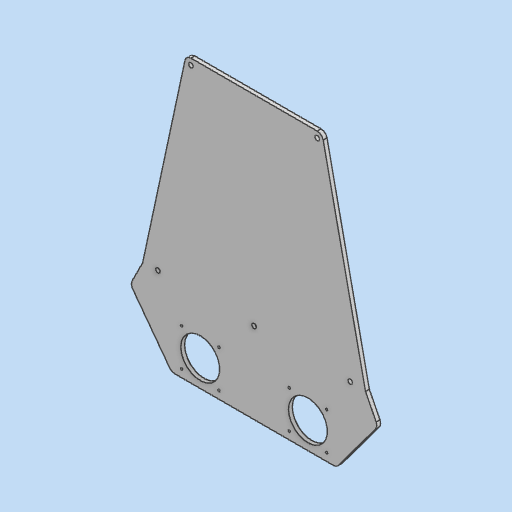
# Autodesk Inventor part: ChestFrontPanel
Saved by Autodesk Inventor 2025.2 (Build 292293000, 293)
## iProperties
Created: 2025-09-23
Part Number: ChestFrontPanel
Material: Generic
Document SubType Name: Sheet Metal
Designer: valer
Density: 1 g/cm^3
Sheet Metal Rule: Default_mm
Appearance: Default
Author: valer
Autodesk Inventor part; units mm, degrees
ref_plane "YZ Plane" through (0, 0, 0) normal (1, 0, 0) x (0, 1, 0)
ref_plane "XZ Plane" through (0, 0, 0) normal (0, 1, 0) x (-1, 0, 0)
ref_plane "XY Plane" through (0, 0, 0) normal (0, 0, 1) x (1, 0, 0)
sketch "Base" plane through (0, 0, 0) normal (0, 0, 1) x (1, 0, 0)
  line L0 (-341.7653, 0) -> (341.7653, 0) construction
  line L1 (0, -75.5138) -> (0, 453.0828) construction
  line L2 (183.676, 264.154) -> (223.6199, 230.6371) construction
  arc A0 (180.154, 267.676) -> (183.676, 264.154) centre (202.0437, 286.0437) ccw construction
  line L3 (105.6111, 356.5128) -> (180.154, 267.676) construction
  arc A1 (105.6111, 356.5128) -> (69.1282, 373.525) centre (69.1282, 325.9) ccw construction
  line L4 (-69.1282, 373.525) -> (69.1282, 373.525) construction
  arc A2 (231.2425, 165.7605) -> (223.6199, 230.6371) centre (193.0071, 194.1542) ccw construction
  line L5 (231.2425, 165.7605) -> (183.8243, 101.9065) construction
  line L6 (0, 373.525) -> (69.1282, 373.525) construction
  line L7 (183.8243, 101.9065) -> (108.1482, 0) construction
  line L8 (-183.676, 264.154) -> (-223.6199, 230.6371) construction
  arc A3 (-183.676, 264.154) -> (-180.154, 267.676) centre (-202.0437, 286.0437) ccw construction
  line L9 (-105.6111, 356.5128) -> (-180.154, 267.676) construction
  arc A4 (-69.1282, 373.525) -> (-105.6111, 356.5128) centre (-69.1282, 325.9) ccw construction
  arc A5 (-223.6199, 230.6371) -> (-231.2425, 165.7605) centre (-193.0071, 194.1542) ccw construction
  line L10 (-231.2425, 165.7605) -> (-183.8243, 101.9065) construction
  line L11 (0, 373.525) -> (-69.1282, 373.525) construction
  line L12 (-183.8243, 101.9065) -> (-108.1482, 0) construction
  line L13 (108.1482, 0) -> (-108.1482, 0)
  line L14 (-108.1482, 0) -> (-186.1215, 105)
  line L15 (-186.1215, 105) -> (186.1215, 105)
  line L16 (186.1215, 105) -> (108.1482, 0)
  point P0 (0, 105)
extrude "Plate1" add sketch "Base" along normal blind 5
chamfer "SideChamferFeature" distance 40 angle 45 2 edges at (-186.1215, 105, 2.5) (186.1215, 105, 2.5)
fillet "OutsideFillets1Feature" radius 8 4 edges at (108.1482, 0, 2.5) (162.2738, 72.8863, 2.5) (-108.1482, 0, 2.5) (-162.2738, 72.8863, 2.5)
sketch "Mount" plane through (0, 0, 0) normal (0, 0, -1) x (-1, 0, 0)
  line L0 (-146.1215, 105) -> (146.1215, 105)
  line L1 (-146.1215, 105) -> (-89.2554, 369.0629)
  line L2 (0, -75.5138) -> (0, 453.0828) construction
  line L3 (-89.2554, 369.0629) -> (0, 369.0629)
  arc A0 (-69.1282, 373.525) -> (-105.6111, 356.5128) centre (-69.1282, 325.9) ccw construction
  line L4 (146.1215, 105) -> (89.2554, 369.0629)
  line L5 (89.2554, 369.0629) -> (0, 369.0629)
  point P0 (0, 0)
sheet face with bend "MountFeature" sketch "Mount" thickness 5 toward (0, 0, 1) bend radius 5 relief straight relief width 5 relief depth 2.5
bend "Bend1"
fillet "TopFilletsFeature" radius 8 2 edges at (89.2554, 369.0629, 2.5) (-89.2554, 369.0629, 2.5)
sketch "FrameMount" plane through (0, 0, 0) normal (0, 0, -1) x (-1, 0, 0)
  arc A0 (-82.7948, 369.0629) -> (-90.6155, 362.7471) centre (-82.7948, 361.0629) ccw construction
  circle A1 centre (-82.7948, 361.0629) radius 3
  line L0 (-87.8211, 367.2868) -> (-82.7948, 361.0629) construction
  line L1 (0, -74.0889) -> (0, 444.5336) construction
  circle A2 centre (-126.1215, 106.2592) radius 3
  line L2 (-146.1215, 105) -> (-160.0581, 77.2916) construction
  circle A3 centre (82.7948, 361.0629) radius 3
  circle A4 centre (126.1215, 106.2592) radius 3
  line L3 (-126.1215, 106.2592) -> (126.1215, 106.2592) construction
  circle A5 centre (0, 106.2592) radius 3
  point P0 (0, 0)
  dimension "d44" = 6
  dimension "d45" = 8
  dimension "d47" = 6
  dimension "d56" = 20
  constraints: 5 centre point, 4 end point, 2 point on circle, 2 symmetric about line, 1 coincident, 1 equal radius, 1 horizontal, 1 midpoint, 1 point on line, 2 other
  measures "d44" diameter of A1
  measures "d45" distance of A1.centre point (-87.821, 367.287)
  measures "d47" diameter of A2
  measures "d56" horizontal distance of A2.centre L2.start
extrude "FrameMountHolesFeature" cut sketch "FrameMount" against normal blind 5
sketch "ExternalHoles" plane through (0, 0, 0) normal (0, 0, -1) x (-1, 0, 0)
  circle A0 centre (20, 67) radius 2.7 projected
  circle A1 centre (20, 85) radius 2.7 projected
  circle A2 centre (-20, 67) radius 2.7 projected
  circle A3 centre (-20, 85) radius 2.7 projected
  circle A4 centre (95.1, 10) radius 1.5 projected
  circle A5 centre (70.6, 34.5) radius 25.5 projected
  circle A6 centre (95.1, 59) radius 1.5 projected
  circle A7 centre (46.1, 59) radius 1.5 projected
  circle A8 centre (46.1, 10) radius 1.5 projected
  circle A9 centre (-70.6, 34.5) radius 25.5 projected
  circle A10 centre (-95.1, 10) radius 1.5 projected
  circle A11 centre (-46.1, 10) radius 1.5 projected
  circle A12 centre (-95.1, 59) radius 1.5 projected
  circle A13 centre (-46.1, 59) radius 1.5 projected
  point P0 (0, 0)
extrude "Cut4" cut sketch "ExternalHoles" against normal blind 5 contours A4 | A5 | A6 | A7 | A8 | A9 | A10 | A11 | A12 | A13
equation "\"d48\" = Thickness"
equation "\"d0\" = Thickness"
equation "\"d17\" = BendRadius"
equation "\"d18\" = BendReliefWidth"
equation "\"d20\" = MinimumRemnant"
equation "\"d19\" = BendReliefDepth"
equation "\"d21\" = TransitionRadius"
equation "\"BendRadius\" = Thickness"
equation "\"BendReliefWidth\" = Thickness"
equation "\"BendReliefDepth\" = 0.5 * Thickness"
equation "\"TransitionRadius\" = BendRadius"
equation "\"JacobiRadiusSize\" = BendRadius"
equation "\"GapSize\" = Thickness"
equation "\"Thickness\" = 5"
equation "\"MinimumRemnant\" = 10"
body "Solid1"
